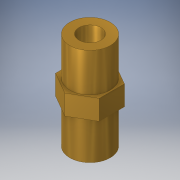
# Autodesk Inventor part: am-2187
Saved by Autodesk Inventor 2016 SP2 (Build 200236200, 236)
## iProperties
Created: 2017-03-28
Part Number: am-2187
Material: Brass
Document SubType Name: Modeling
Designer: smiku
Mass: 13.3574 g
Surface Area: 14.3371 cm^2
Volume: 1.57331 cm^3
Density: 8.49 g/cm^3
Appearance: Brass - Polished
Author: smiku
Autodesk Inventor part; units mm, degrees
ref_plane "YZ Plane" through (0, 0, 0) normal (1, 0, 0) x (0, 1, 0)
ref_plane "XZ Plane" through (0, 0, 0) normal (0, 1, 0) x (-1, 0, 0)
ref_plane "XY Plane" through (0, 0, 0) normal (0, 0, 1) x (1, 0, 0)
sketch "Sketch1" plane through (0, 0, 0) normal (0, 1, 0) x (-1, 0, 0)
  circle A0 centre (0, 0) radius 5.5499 construction
  line L0 (5.5499, -3.2042) -> (0, -6.4085)
  line L1 (0, -6.4085) -> (-5.5499, -3.2042)
  line L2 (-5.5499, -3.2042) -> (-5.5499, 3.2042)
  line L3 (-5.5499, 3.2042) -> (0, 6.4085)
  line L4 (0, 6.4085) -> (5.5499, 3.2042)
  line L5 (5.5499, 3.2042) -> (5.5499, -3.2042)
  circle A1 centre (0, 0) radius 2.8067
  circle A2 centre (0, 0) radius 5.1562
  point P0 (5.5499, 0)
  dimension "d0" = 11.0998
  dimension "d1" = 5.6134
  dimension "d4" = 10.3124
  constraints: 12 end point, 4 coincident, 2 centre point, 1 horizontal alignment, 1 midpoint, 1 vertical, 15 other
  measures "d1" diameter of A1
  measures "d4" diameter of A2
extrude "Extrusion1" add sketch "Sketch1" along normal mid plane 5.08 contours L0 L1 L2 L3 L4 L5 | A2
extrude "Extrusion2" add sketch "Sketch1" along normal mid plane 24.765 contours A2
body "Solid1"
